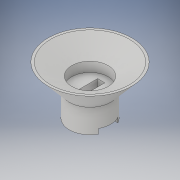
# Autodesk Inventor part: fitted nu funnel easy angle
Saved by Autodesk Inventor 2019 (Build 230136000, 136)
## iProperties
Created: 2020-09-26
Part Number: fitted nu funnel easy angle
Material: Generic
Document SubType Name: Modeling
Designer: Obscure_Decision
Density: 1 g/cm^3
Appearance: Default
Author: Obscure_Decision
Autodesk Inventor part; units mm, degrees
ref_plane "YZ Plane" through (0, 0, 0) normal (1, 0, 0) x (0, 1, 0)
ref_plane "XZ Plane" through (0, 0, 0) normal (0, 1, 0) x (-1, 0, 0)
ref_plane "XY Plane" through (0, 0, 0) normal (0, 0, 1) x (1, 0, 0)
sketch "Sketch2" plane through (0, 0, 0) normal (1, 0, 0) x (0, 1, 0)
  line L0 (0, 0) -> (0, -17)
  line L1 (0, 0) -> (22, 0)
  line L2 (22, 0) -> (22, -15)
  line L3 (22, 0) -> (30, 0) construction
  line L4 (30, 0) -> (30, -17) construction
  line L5 (22, -17) -> (22, -15) construction
  line L6 (30, 0) -> (40, 0)
  line L7 (40, 0) -> (40, -34.5) construction
  line L8 (40, -34.5) -> (40, -32.5)
  line L9 (40, -32.5) -> (30, -15)
  line L10 (22, -15) -> (30, -15)
  line L11 (22, -15) -> (22, 0) construction
  line L12 (40, -34.5) -> (19.6496, -17)
  line L13 (19.6496, -17) -> (0, -17)
  dimension "d0" = 17
  dimension "d1" = 22
  dimension "d3" = 8
  dimension "d4" = 10
  dimension "d5" = 34.5
  dimension "d6" = 2
  constraints: 28 end point, 3 perpendicular, 3 point on line, 2 horizontal, 2 parallel, 1 vertical
  measures "d0" distance of L0.start L0.end
  measures "d1" distance of L0.start L1.end
  measures "d3" distance of L4.end L5.start
  measures "d4" distance of L3.end L6.end
  measures "d5" distance of L6.end L7.end
  measures "d6" distance of L7.end L8.end
revolve "Revolution1" add sketch "Sketch2" angle 360 about axis through (0, 22, 0) along (0, 1, 0)
sketch "Sketch3" plane through (0, 22, 0) normal (0, 1, 0) x (1, 0, 0)
  line L0 (-3, -9.275) -> (3, -9.275)
  line L1 (3, -9.275) -> (3, 9.275)
  line L2 (3, 9.275) -> (-3, 9.275)
  line L3 (-3, 9.275) -> (-3, -9.275)
  line L4 (-3, -9.275) -> (3, 9.275) construction
  line L5 (3, -9.275) -> (-3, 9.275) construction
  point P0 (0, 0)
  dimension "d8" = 6
  dimension "d9" = 18.55
  constraints: 12 end point, 2 midpoint, 2 parallel, 1 horizontal, 1 perpendicular
  measures "d8" distance of L2.end L1.end
  measures "d9" distance of L1.end L0.end
extrude "Extrusion1" cut sketch "Sketch3" against normal blind 15
sketch "Sketch4" plane through (0, 7, 0) normal (0, 1, 0) x (1, 0, 0)
  line L0 (-1.5, -8) -> (1.5, -8)
  line L1 (1.5, -8) -> (1.5, 8)
  line L2 (1.5, 8) -> (-1.5, 8)
  line L3 (-1.5, 8) -> (-1.5, -8)
  line L4 (-1.5, -8) -> (1.5, 8) construction
  line L5 (1.5, -8) -> (-1.5, 8) construction
  point P0 (0, 0)
  dimension "d12" = 3
  dimension "d13" = 16
  constraints: 12 end point, 2 midpoint, 2 parallel, 1 horizontal, 1 perpendicular
  measures "d12" distance of L2.end L1.end
  measures "d13" distance of L1.end L0.end
extrude "Extrusion2" cut sketch "Sketch4" against normal blind 7
sketch "Sketch5" plane through (0, 0, 0) normal (0, -1, 0) x (1, 0, 0)
  line L0 (1.5, -8) -> (1.5, 8) projected
  line L1 (1.5, -8) -> (17.518, -8)
  line L2 (17.518, -8) -> (17.518, 8)
  line L3 (17.518, 8) -> (1.5, 8)
  line L4 (1.5, 8) -> (1.5, -8)
  point P0 (0, 0)
  constraints: 8 end point, 2 parallel, 1 horizontal, 1 perpendicular
extrude "Extrusion3" cut sketch "Sketch5" against normal blind 4
body "Solid1"
